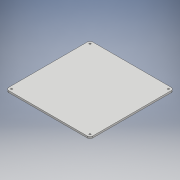
# Autodesk Inventor part: SheetPot
Saved by Autodesk Inventor 2018 (Build 220112000, 112)
## iProperties
Created: 2019-06-03
Part Number: SheetPot
Material: Generic
Document SubType Name: Modeling
Designer: aal_9
Density: 1 g/cm^3
Appearance: Default
Author: aal_9
Autodesk Inventor part; units mm, degrees
ref_plane "YZ Plane" through (0, 0, 0) normal (1, 0, 0) x (0, 1, 0)
ref_plane "XZ Plane" through (0, 0, 0) normal (0, 1, 0) x (-1, 0, 0)
ref_plane "XY Plane" through (0, 0, 0) normal (0, 0, 1) x (1, 0, 0)
sketch "Sketch1" plane through (0, 0, 0) normal (0, 0, 1) x (1, 0, 0)
  line L0 (-70, 70.3846) -> (80, 70.3846)
  line L1 (80, 70.3846) -> (80, -79.6154)
  line L2 (80, -79.6154) -> (-70, -79.6154)
  line L3 (-70, -79.6154) -> (-70, 70.3846)
  point P0 (0, 0)
  dimension "d0" = 150
  dimension "d1" = 150
  constraints: 8 end point, 2 parallel, 1 horizontal, 1 perpendicular
  measures "d0" distance of L0.start L0.end
  measures "d1" distance of L2.end L0.start
extrude "Extrusion1" add sketch "Sketch1" along normal blind 3.175
sketch "Sketch2" plane through (0, 0, 3.175) normal (0, 0, 1) x (1, 0, 0)
  line L0 (80, 70.3846) -> (-70, 70.3846) projected
  line L1 (-70, 70.3846) -> (-70, -79.6154) projected
  line L2 (80, -79.6154) -> (80, 70.3846) projected
  line L3 (-70, -79.6154) -> (80, -79.6154) projected
  point P0 (0, 0)
  point P1 (-65, 65.3846)
  point P2 (75, 65.3846)
  point P3 (75, -74.6154)
  point P4 (-65, -74.6154)
  dimension "d4" = 5
  dimension "d5" = 5
  dimension "d6" = 5
  dimension "d7" = 5
  dimension "d8" = 5
  dimension "d9" = 5
  dimension "d10" = 5
  dimension "d11" = 5
  measures "d4" distance from line of L0 point (-65, 65.385)
  measures "d5" distance from line of L1 point (-65, 65.385)
  measures "d6" distance from line of L0 point (75, 65.385)
  measures "d7" distance from line of L2 point (75, 65.385)
  measures "d8" distance from line of L3 point (-65, -74.615)
  measures "d9" distance from line of L1 point (-65, -74.615)
  measures "d10" distance from line of L2 point (75, -74.615)
  measures "d11" distance from line of L3 point (75, -74.615)
hole "Hole1" at (-65, 65.3846, 3.175) at (75, 65.3846, 3.175) at (75, -74.6154, 3.175) at (-65, -74.6154, 3.175) direction (0, 0, -1) diameter 3 end through all
fillet "Fillet1" radius 5 4 edges at (-70, 70.3846, 1.5875) (80, 70.3846, 1.5875) (80, -79.6154, 1.5875) (-70, -79.6154, 1.5875)
body "Solid1"
